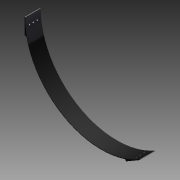
# Autodesk Inventor part: 120 degree curved track
Saved by Autodesk Inventor 2011 SP1 (Build 150282100, 282)
## iProperties
Created: 2013-01-18
Part Number: 120 degree curved track
Document SubType Name: Modeling
Designer: wes
Density: 1 g/cm^3
Author: wes
Autodesk Inventor part; units mm, degrees
ref_plane "YZ Plane" through (0, 0, 0) normal (1, 0, 0) x (0, 1, 0)
ref_plane "XZ Plane" through (0, 0, 0) normal (0, 1, 0) x (-1, 0, 0)
ref_plane "XY Plane" through (0, 0, 0) normal (0, 0, 1) x (1, 0, 0)
sketch "Sketch1" plane through (0, 0, 0) normal (0, 0, 1) x (1, 0, 0)
  arc A0 (-375.92, 0) -> (187.96, -325.5563) centre (0, 0) ccw
  arc A1 (-378.46, 0) -> (189.23, -327.756) centre (0, 0) ccw
  line L0 (0, 0) -> (189.23, -327.756)
  line L1 (0, 0) -> (-378.46, 0)
  line L2 (-378.46, 0) -> (-378.46, -78.74)
  line L3 (-378.46, -78.74) -> (-370.1783, -78.74)
  line L4 (189.23, -327.756) -> (121.0392, -367.126)
  line L5 (121.0392, -367.126) -> (116.8983, -359.9538)
  dimension "d0" = 751.84
  dimension "d1" = 756.92
  dimension "d2" = 120
  dimension "d3" = 78.74
  dimension "d4" = 78.74
  constraints: 12 end point, 6 point on circle, 4 perpendicular, 2 centre point, 2 coincident, 2 point on line, 2 tangent, 1 horizontal
  measures "d0" diameter of A0
  measures "d1" diameter of A1
  measures "d2" angle of L0 L1
  measures "d3" distance of L1.end L2.end
  measures "d4" distance of L0.end L4.end
extrude "Extrusion1" add sketch "Sketch1" along normal blind 76.2 contours A0 L0 A1 L1 | A1 L3 L2 | L4 L5 A1
sketch "Sketch2" plane through (121.0392, -367.126, 0) normal (0.5, -0.866, 0) x (0.866, 0.5, 0)
  line L0 (0, 0) -> (78.74, 0) projected
  line L1 (78.74, 0) -> (78.74, 76.2) projected
  point P0 (39.37, 19.05)
  point P1 (39.37, 38.1)
  point P2 (39.37, 57.15)
  dimension "d7" = 19.05
  dimension "d8" = 38.1
  dimension "d9" = 57.15
  dimension "d10" = 39.37
  dimension "d11" = 39.37
  dimension "d12" = 39.37
  measures "d7" distance from line of L0 point (39.37, 19.05)
  measures "d8" distance from line of point (39.37, 38.1) L0
  measures "d9" distance from line of point (39.37, 57.15) L0
  measures "d10" distance from line of L1 point (39.37, 19.05)
  measures "d11" distance from line of L1 point (39.37, 38.1)
  measures "d12" distance from line of L1 point (39.37, 57.15)
sketch "Sketch3" plane through (-378.46, -78.74, 0) normal (-1, 0, 0) x (0, 0, 1)
  line L0 (0, 78.74) -> (76.2, 78.74) projected
  line L1 (0, 78.74) -> (0, 0) projected
  point P0 (19.05, 39.37)
  point P1 (38.1, 39.37)
  point P2 (57.15, 39.37)
  dimension "d13" = 19.05
  dimension "d14" = 38.1
  dimension "d15" = 57.15
  dimension "d16" = 39.37
  dimension "d17" = 39.37
  dimension "d18" = 39.37
  measures "d13" distance from line of L1 point (19.05, 39.37)
  measures "d14" distance from line of point (38.1, 39.37) L1
  measures "d15" distance from line of point (57.15, 39.37) L1
  measures "d16" distance from line of L0 point (19.05, 39.37)
  measures "d17" distance from line of L0 point (38.1, 39.37)
  measures "d18" distance from line of L0 point (57.15, 39.37)
hole "Hole1" at (-378.46, -39.37, 57.15) at (-378.46, -39.37, 38.1) at (-378.46, -39.37, 19.05) direction (1, 0, 0) diameter 6.35 depth 25.4 tip angle 118
hole "Hole2" at (155.1346, -347.441, 19.05) at (155.1346, -347.441, 38.1) at (155.1346, -347.441, 57.15) direction (-0.5, 0.866, 0) diameter 6.35 depth 25.4 tip angle 118
body "Solid1"
